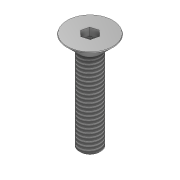
# Autodesk Inventor part: Tornillo Allen cabeza fresada M4x16mm
Saved by Autodesk Inventor 2020.3 (Build 243373000, 373)
## iProperties
Created: 2020-05-08
Part Number: Tornillo Allen cabeza fresada M4x16mm
Material: Generic
Document SubType Name: Modeling
Designer: Dante
Density: 1 g/cm^3
Appearance: Rubber - Black - Version 1.1
Mass: 0.242439 g
Surface Area: 2.80465 cm^2
Volume: 0.242439 cm^3
Author: Dante
Autodesk Inventor part; units mm, degrees
ref_plane "YZ Plane" through (0, 0, 0) normal (1, 0, 0) x (0, 1, 0)
ref_plane "XZ Plane" through (0, 0, 0) normal (0, 1, 0) x (-1, 0, 0)
ref_plane "XY Plane" through (0, 0, 0) normal (0, 0, 1) x (1, 0, 0)
sketch "Sketch1" plane through (0, 0, 0) normal (0, 0, 1) x (1, 0, 0)
  line L0 (-14.4028, -27.52) -> (-9.9228, -27.52)
  line L1 (-9.9228, -27.52) -> (-9.9228, -31)
  line L2 (-9.9228, -31) -> (-9.9228, -46)
  line L3 (-9.9228, -46) -> (-11.9228, -46)
  line L4 (-11.9228, -46) -> (-11.9228, -30)
  line L5 (-11.9228, -30) -> (-14.4028, -27.52)
  point P0 (0, 0)
  dimension "d3" = 2
  dimension "d15" = 2.48
  dimension "d16" = 4.48
  dimension "d24" = 90
  dimension "d25" = 16
  constraints: 12 end point, 2 perpendicular, 2 vertical
  measures "d3" distance of L2.end L3.end
  measures "d15" distance from line of L0 L4.end
  measures "d16" distance of L0.end L0.start
  measures "d24" angle of L1 L0
  measures "d25" distance of L3.end L4.end
revolve "Revolution1" add sketch "Sketch1" angle 360 about axis through (-9.9228, -31, 0) along (0, -1, 0)
chamfer "Chamfer2" distance 0.2 angle 45 1 edges at (-7.9228, -46, 0)
thread "Rosca1" size "M4x0.7" class "6g" standard "ANSI Metric M Profile" full length
chamfer "Chaflán3" distance 0.2 angle 45 1 edges at (-5.4428, -27.52, 0)
sketch "Boceto2" plane through (-9.9228, -27.52, 0) normal (0, 1, 0) x (1, 0, 0)
  line L0 (-1.0464, 0.9942) -> (0.3378, 1.4033)
  line L1 (0.3378, 1.4033) -> (1.3842, 0.4091)
  line L2 (1.3842, 0.4091) -> (1.0464, -0.9942)
  line L3 (1.0464, -0.9942) -> (-0.3378, -1.4033)
  line L4 (-0.3378, -1.4033) -> (-1.3842, -0.4091)
  line L5 (-1.3842, -0.4091) -> (-1.0464, 0.9942)
  point P0 (9.9228, 0)
  point P1 (0, 0)
  dimension "d20" = 2.5
  constraints: 12 end point, 13 other
  measures "d20" distance between parallel lines of L1 L4
extrude "Extrusión1" cut sketch "Boceto2" against normal blind 1.5
body "Solid1"
